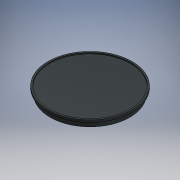
# Autodesk Inventor part: 下
Saved by Autodesk Inventor 2017 (Build 210142000, 142)
## iProperties
Part Number: 下
Material: SS41
Document SubType Name: Modeling
Designer: G
Density: 7.85 g/cm^3
Appearance: 鐵灰色
Author: G
Autodesk Inventor part; units mm, degrees
ref_plane "XZ Plane" through (0, 0, 0) normal (0, 1, 0) x (-1, 0, 0)
ref_plane "XY Plane" through (0, 0, 0) normal (0, 0, 1) x (1, 0, 0)
sketch "草圖1" plane through (6.7908, 20.3797, 0) normal (0, 0, -1) x (-1, 0, 0)
  circle A0 centre (-32.1517, 18.5628) radius 37.1256 projected
  point P0 (6.7908, -20.3797)
ref_plane "工作平面1" through (38.9425, 38.9425, 0) normal (1, 0, 0) x (0, 1, 0)
sketch "草圖2" plane through (38.9425, 38.9425, 0) normal (1, 0, 0) x (0, 1, 0)
  line L0 (-38.9425, 0) -> (-38.9425, 6)
  line L1 (-38.9425, 6) -> (-76.4425, 6)
  line L2 (-76.4425, 6) -> (-76.4425, 7)
  line L3 (-76.4425, 7) -> (-77.9425, 7)
  line L4 (-77.9425, 7) -> (-77.9425, 5)
  line L5 (-77.9425, 5) -> (-75.9425, 5)
  line L6 (-75.9425, 5) -> (-75.9425, 0)
  line L7 (-75.9425, 0) -> (-38.9425, 0)
  dimension "d0" = 74
  dimension "d1" = 78
  dimension "d4" = 75
  dimension "d7" = 7
  dimension "d8" = 5
  dimension "d9" = 6
  constraints: 16 end point, 7 perpendicular, 1 coincident, 1 vertical
  measures "d0" diameter of L6 L0
  measures "d1" diameter of L4 L0
  measures "d4" diameter of L2 L0
  measures "d7" distance between parallel lines of L3 L7
  measures "d8" distance between parallel lines of L5 L7
  measures "d9" distance between parallel lines of L7 L1
revolve "迴轉1" add sketch "草圖2" angle 360 about axis through (38.9425, 0, 0) along (0, 0, 1)
